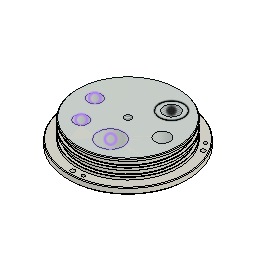
end_cap_drillings_sensors (Autodesk Fusion 360 design; units mm, degrees)
Autodesk Fusion 360 part; units mm, degrees
note: some values were not read from the file. Chosen so that the rebuilt part matches the saved one: which face or edge a step refers to. Set by a fixed rule: which sketch regions a step uses.
sketch "Sketch1" plane through (0, 0, 0) normal (0, 1, 0) x (1, 0, 0)
  line L0 (0, 0) -> (45, 0)
  line L1 (45, 0) -> (45, -5)
  line L2 (45, -5) -> (38, -5)
  line L3 (38, -19) -> (0, -19)
  line L4 (0, -19) -> (0, 0)
  line L5 (38, -7) -> (35.7, -7)
  line L6 (35.7, -7) -> (35.7, -11)
  line L7 (35.7, -11) -> (38, -11)
  line L8 (38, -13) -> (35.7, -13)
  line L9 (35.7, -13) -> (35.7, -17)
  line L10 (35.7, -17) -> (38, -17)
  line L11 (38, -5) -> (38, -7)
  line L12 (38, -11) -> (38, -13)
  line L13 (38, -17) -> (38, -19)
  dimension "d2" = 45
  dimension "d4" = 5
  dimension "d5" = 7
  dimension "d9" = 4
  dimension "d10" = 4
  dimension "d11" = 2.3
  dimension "d13" = 2
  dimension "d14" = 2
  dimension "d15" = 2
  dimension "d16" = 19
  constraint coincident L0.start L4.end
  constraint horizontal L0
  constraint perpendicular L0 L1
  constraint perpendicular L1 L2
  constraint perpendicular L2 L11
  constraint perpendicular L1 L3
  constraint perpendicular L0 L4
  constraint perpendicular L5 L11
  constraint perpendicular L5 L6
  constraint perpendicular L7 L11
  constraint coincident L8.start L11
  constraint perpendicular L8 L11
  constraint perpendicular L8 L9
  constraint coincident L10.end L11
  constraint perpendicular L10 L11
  constraint collinear L11 L12
  constraint coincident L7.end L11
  constraint collinear L6 L9
  constraint collinear L12 L13
  measures "d2" distance of L0.start L0.end
  measures "d4" distance of L0.end L1.end
  measures "d5" distance of L1.end L2.end
  measures "d9" distance of L5.end L6.end
  measures "d10" distance of L8.end L9.end
  measures "d11" distance of L8.start L8.end
  measures "d13" distance of L3.start L10.end
  measures "d14" distance of L7.end L8.start
  measures "d15" distance of L2.end L5.start
  measures "d16" distance of L3.end L0.start
revolve "Revolve1" add sketch "Sketch1" angle 360 about axis through (0, 0, 19) along (0, 0, -1)
chamfer "Chamfer1" distance 1 angle 45 1 edges at (-41.9547, -16.2727, 0)
chamfer "Chamfer2" distance 0.5 angle 45 1 edges at (-35.4284, -13.7414, 19)
fillet "Fillet1" radius 0.2 4 edges at (-35.4284, -13.7414, 17) (-35.4284, -13.7414, 13) (-35.4284, -13.7414, 11) (-35.4284, -13.7414, 7)
fillet "Fillet2" radius 0.3 2 faces at (35.6556, 1.7795, 14.3333) (35.6556, 1.7795, 8.3333)
chamfer "Chamfer7" distance 0.5 angle 45 1 edges at (-41.9547, -16.2727, 5)
sketch "Sketch5" plane through (0, 0, 0) normal (0, 0, -1) x (1, 0, 0)
  circle A0 centre (0, 0) radius 44
  line L0 (1.75, 0) -> (22.5, 0)
  circle A1 centre (12, -20.7846) radius 5.7
  circle A2 centre (12, -20.7846) radius 12.7
  circle A3 centre (0, 0) radius 38
  line L1 (0, 0) -> (12, -20.7846)
  circle A4 centre (26, 0) radius 5.65
  line L2 (0, 0) -> (26, 0) construction
  circle A5 centre (26, 0) radius 13.5
  circle A6 centre (0, 0) radius 45
  circle A7 centre (26, 0) radius 10
  circle A8 centre (-25, 0) radius 5.1
  line L3 (0, 0) -> (-25, 0)
  circle A9 centre (-25, 0) radius 9.5
  circle A10 centre (0, 0) radius 35.7
  circle A11 centre (0, 0) radius 35.7
  circle A12 centre (0, 0) radius 35.7
  circle A13 centre (0, 0) radius 35.7
  circle A14 centre (7.5244, 20.6732) radius 9.5
  circle A15 centre (-16.0697, 19.1511) radius 5.1
  line L4 (29.9224, -40.4151) -> (37.1692, -40.4151) construction
  line L5 (37.1692, -40.4151) -> (37.1692, -37.2529) construction
  line L6 (37.1692, -37.2529) -> (29.9224, -37.2529) construction
  line L7 (29.9224, -37.2529) -> (29.9224, -40.4151) construction
  line L8 (48.7898, 4.4749) -> (58.5942, 4.4749) construction
  line L9 (58.5942, 4.4749) -> (58.5942, 9.0817) construction
  line L10 (58.5942, 9.0817) -> (48.7898, 9.0817) construction
  line L11 (48.7898, 9.0817) -> (48.7898, 4.4749) construction
  line L12 (23.0567, 44.7996) -> (29.6447, 44.7996) construction
  line L13 (29.6447, 44.7996) -> (29.6447, 47.9619) construction
  line L14 (29.6447, 47.9619) -> (23.0567, 47.9619) construction
  line L15 (23.0567, 47.9619) -> (23.0567, 44.7996) construction
  line L16 (-58.4122, 26.6088) -> (-42.3374, 26.6088) construction
  line L17 (-42.3374, 26.6088) -> (-42.3374, 30.8251) construction
  line L18 (-42.3374, 30.8251) -> (-58.4122, 30.8251) construction
  line L19 (-58.4122, 30.8251) -> (-58.4122, 26.6088) construction
  circle A16 centre (7.5244, 20.6732) radius 12
  circle A17 centre (-16.0697, 19.1511) radius 9.5
  circle A18 centre (0, 0) radius 31.7 construction
  point P0 (0, 41.5)
  point P1 (7.2064, 40.8695)
  dimension "d78" = 25.4
  dimension "d79" = 11.4
  dimension "d89" = 24
  dimension "d99" = 27
  dimension "d100" = 11.3
  dimension "d102" = 41.5
  dimension "d103" = 41.5
  dimension "d104" = 10
  dimension "d116" = 20
  dimension "d118" = 25
  dimension "d121" = 26
  dimension "d139" = 19
  dimension "d140" = 3
  dimension "d141" = 3
  dimension "d142" = 3
  dimension "d143" = 3
  dimension "d144" = 22
  dimension "d145" = 24
  dimension "d146" = 70
  dimension "d148" = 10.2
  dimension "d149" = 19
  dimension "d150" = 25
  dimension "d151" = 60
  dimension "d152" = 50
  dimension "d160" = 4
  dimension "d161" = 120
  constraint concentric A1 A2
  constraint coincident A0.centre A3.centre
  constraint coincident A1.centre A2.centre
  constraint coincident A4.centre L2.end
  constraint concentric A4 A5
  constraint concentric A4 A7
  constraint coincident A8.centre L3.end
  constraint concentric A8 A9
  constraint vertical A0.centre P0
  constraint coincident L0 A4.centre
  constraint concentric A14 A16
  constraint concentric A15 A17
  constraint equal A8 A15
  constraint equal A9 A17
  measures "d78" diameter of A2
  measures "d79" diameter of A1
  measures "d89" distance of A0.centre A1.centre
  measures "d99" diameter of A5
  measures "d100" diameter of A4
  measures "d102" distance of A0.centre P0
  measures "d103" distance of A0.centre P1
  measures "d104" angle of A0.centre P0 P1
  measures "d116" diameter of A7
  measures "d118" distance of A0.centre A8.centre
  measures "d121" distance of A0.centre A4.centre
  measures "d139" diameter of A14
  measures "d144" distance of A0.centre A14.centre
  measures "d145" diameter of A16
  measures "d146" angle of A0.centre A4.centre A14.centre
  measures "d148" diameter of A15
  measures "d149" diameter of A17
  measures "d150" distance of A0.centre A15.centre
  measures "d151" angle of A0.centre A15.centre A14.centre
  measures "d152" angle of A0.centre A8.centre A15.centre
  measures "d160" distance of A11 A18
  measures "d161" angle of A1.centre A0.centre A8.centre
hole "Hole8" at (12, 20.7846, 0) direction (0, 0, 1) diameter 11 end through all
thread "Thread5" "BSP Pipe Threads 1/4 G 1/4-19" major diameter 13.157 minor diameter 11.6675 pitch 1.3368 angle 55 resizes the face on face at (12.2742, 26.2778, 6.3333)
hole "Hole10" at (0, 0, 19) direction (0, 0, -1) diameter 5.035 depth 9 tip angle 118
thread "Thread6" "ISO Metric profile 6.0 M6x1 6H" thread offset 0 thread depth 8
hole "Hole11" at (0, -41.5, 0) direction (0, 0, 1) diameter 3.2 end through all
hole "Hole12" at (7.2064, -40.8695, 0) direction (0, 0, 1) diameter 2.529 end through all
thread "Thread7" "ISO Metric profile 3.0 M3x0.5 6H" thread offset 0 thread depth 10
pattern_circular "C-Pattern3" count 3 over 360 about axis through (0, 0, 1.75) along (0, 0, 1) of "Hole11", "Hole12"
extrude "Extrude1" cut sketch "Sketch5" against normal blind 20 contours A4
extrude "Extrude2" cut sketch "Sketch5" against normal blind 27 contours A8 | A15
extrude "Extrude6" cut sketch "Sketch5" against normal blind 4 contours A9 | A17
extrude "Extrude7" cut sketch "Sketch5" against normal through all contours A14
chamfer "Chamfer10" distance 0.5 angle 45 4 edges at (-29.7549, 1.8442, 4) (-20.8246, -17.3069, 4) (-1.3327, -24.1086, 0) (20.7324, -2.0431, 0)
extrude "Extrude3" cut sketch "Sketch5" against normal blind 0.01 contours L0 A5 A7 A10 A11 A12 A13 | L0 A2 A5 A7 A10 A11 A12 A13 | A7 A10 A11 A12 A13 | A3 A5 A7 A10 A11 A12 A13 | A2 A5 | A7 A10 A11 A12 A13 | A3 A5 | A16
sketch "Sketch6" plane through (0, 0, 19) normal (0, 0, 1) x (-1, 0, 0)
  circle A0 centre (0, 0) radius 37.5
  circle A1 centre (-12, -20.7846) radius 5.8338
  circle A2 centre (0, 0) radius 2.5175
  circle A3 centre (-26, 0) radius 5.65
  circle A4 centre (-12, -20.7846) radius 9
  circle A5 centre (25, 0) radius 5.1
  circle A6 centre (16.0697, 19.1511) radius 5.1
  circle A7 centre (-7.5244, 20.6732) radius 9.5
  dimension "d132" = 18
  constraint concentric A1 A4
  measures "d132" diameter of A4
extrude "Extrude5" cut sketch "Sketch6" against normal blind 0.01 contours A4
ref_plane "WorkPlane2" through (0, 0, 12.125) normal (-0.173648, -0.984808, 0) x (0, 0, 1)
equation "D_i = 76 mm" comment "Inner Diameter of Cylinder"
equation "d2 = ( D_i + 2 * t ) / 2"
equation "t = 7 mm" comment "Thickness of cylinder wall"
equation "d5 = t"
equation "Oring_depth = 2.3 mm" comment "Depth of Oring Groove"
equation "Oring_width = 4 mm" comment "Width of Oring Groove"
equation "d9 = Oring_width"
equation "d10 = Oring_width"
equation "d11 = Oring_depth"
equation "d102 = ( D_i ) / 2 + t / 2"
equation "d103 = d102"
